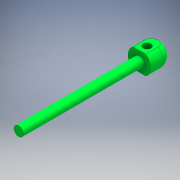
# Autodesk Inventor part: Asta cassetto
Saved by Autodesk Inventor 2016 (Build 200138000, 138)
## iProperties
Created: 2016-09-10
Part Number: Asta cassetto
Material: Generic
Document SubType Name: Modeling
Designer: Muhammad
Density: 1 g/cm^3
Appearance: Default
Author: Muhammad
Autodesk Inventor part; units mm, degrees
ref_plane "YZ Plane" through (0, 0, 0) normal (1, 0, 0) x (0, 1, 0)
ref_plane "XY Plane" through (0, 0, 0) normal (0, 0, 1) x (1, 0, 0)
sketch "Sketch1" plane through (0, 0, 0) normal (0, 1, 0) x (-1, 0, 0)
  circle A0 centre (0, 0) radius 6
  dimension "d0" = 12
  constraints: 1 centre point, 1 coincident
  measures "d0" diameter of A0
extrude "Extrusion1" add sketch "Sketch1" along normal blind 11.5
fillet "Fillet1" radius 5 1 edges at (6, 11.5, 0)
sketch "Sketch2" plane through (0, 0, 0) normal (0, -1, 0) x (1, 0, 0)
  circle A0 centre (0, 0) radius 2.5
  dimension "d4" = 5
  constraints: 1 centre point, 1 coincident
  measures "d4" diameter of A0
extrude "Extrusion2" add sketch "Sketch2" along normal blind 63.5
sketch "Sketch3" plane through (0, 0, 0) normal (0, -1, 0) x (1, 0, 0)
  circle A0 centre (0, 0) radius 2.5 construction
  line L0 (0, -5) -> (0, 5) construction
  circle A1 centre (0, 0) radius 6 projected
  line L1 (-3.3166, -5) -> (3.3166, -5)
  line L2 (-3.3166, 5) -> (3.3166, 5)
  dimension "d8" = 10
  constraints: 6 end point, 4 point on circle, 1 horizontal, 1 parallel
  measures "d8" distance of L0.start L0.end
extrude "Extrusion3" cut sketch "Sketch3" against normal through all contours L2 A1 | A1 L1
sketch "Sketch4" plane through (3.3166, 0, -5) normal (0, 0, -1) x (-1, 0, 0)
  line L0 (3.3166, 0) -> (3.3166, 4) construction
  circle A0 centre (3.3166, 4) radius 2
  dimension "d11" = 4
  constraints: 2 end point, 1 centre point, 1 coincident, 1 vertical
  measures "d11" distance of L0.start L0.end
extrude "Extrusion4" cut sketch "Sketch4" against normal through all
ref_plane "Work Plane1" through (0, 11.5, 0) normal (0, 1, 0) x (-1, 0, 0)
sketch "Sketch5" plane through (0, 11.5, 0) normal (0, 1, 0) x (-1, 0, 0)
  circle A0 centre (0, 0) radius 1.5
  constraints: 1 centre point, 1 coincident
extrude "Extrusion5" cut sketch "Sketch5" against normal up to surface
body "Solid1"
